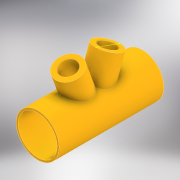
# Autodesk Inventor part: JuntaEjeCadera
Saved by Autodesk Inventor 2021 (Build 250183000, 183)
## iProperties
Created: 2024-02-21
Part Number: JuntaEjeCadera
Material: PLA
Document SubType Name: Modeling
Designer: Martin
Density: 1.27 g/cm^3
Appearance: PLA
Mass: 57.2544 g
Surface Area: 319.514 cm^2
Volume: 45.0822 cm^3
Author: Martin
Autodesk Inventor part; units mm, degrees
ref_plane "YZ Plane" through (0, 0, 0) normal (1, 0, 0) x (0, 1, 0)
ref_plane "XZ Plane" through (0, 0, 0) normal (0, 1, 0) x (-1, 0, 0)
ref_plane "XY Plane" through (0, 0, 0) normal (0, 0, 1) x (1, 0, 0)
sketch "Sketch1" plane through (0, 0, 0) normal (0, 0, 1) x (1, 0, 0)
  circle A0 centre (0, 0) radius 18.6
  circle A1 centre (0, 0) radius 20.5
  dimension "d0" = 37.2
  dimension "d1" = 41
  constraints: 2 centre point, 2 coincident
  measures "d0" diameter of A0
  measures "d1" diameter of A1
extrude "Extrusion1" add sketch "Sketch1" along normal blind 30
ref_plane "Work Plane1" through (0, 0, 0) normal (0, 1, 0) x (0, 0, 1)
ref_plane "Work Plane2" through (0, 40.5, 0) normal (0, 1, 0) x (0, 0, 1)
sketch "Sketch3" plane through (0, 0, 30) normal (0, 0, 1) x (1, 0, 0)
  circle A0 centre (0, 0) radius 20.5 projected
  circle A1 centre (0, 0) radius 18.6 projected
extrude "Extrusion3" add sketch "Sketch3" along normal blind 12
ref_plane "Work Plane3" through (0, 20.5, 0) normal (0, 1, 0) x (-1, 0, 0)
sketch "Sketch5" plane through (0, 40.5, 0) normal (0, 1, 0) x (0, 0, 1)
  line L0 (0, -20.5) -> (0, 20.5) projected
  line L1 (20, 20.5) -> (20, -20.5)
  point P0 (0, 0)
  dimension "d29" = 20
  constraints: 2 end point, 1 vertical
  measures "d29" distance between parallel lines of L0 L1
ref_plane "Work Plane4" through (20.5, 40.5, 20) normal (0, 0.9396926, 0.3420201) x (-1, 0, 0)
sketch "Sketch8" plane through (20.5, 40.5, 20) normal (0, 0.9396926, 0.3420201) x (-1, 0, 0)
  circle A0 centre (20.5, -1.2567) radius 12.5
  circle A1 centre (20.5, -1.2567) radius 7.9
  point P0 (20.5, -4.942)
  dimension "d44" = 25
  dimension "d45" = 15.8
  constraints: 2 centre point, 1 coincident
  measures "d44" diameter of A0
  measures "d45" diameter of A1
extrude "Extrusion6" add sketch "Sketch8" against normal up to surface round surface about axis through (0, 0, 0) along (0, 0, 1) radius 20.5 far side no
mirror "Mirror3" about plane through (0, 0, 0) normal (0, 0, 1) of "Extrusion1", "Extrusion6", "Extrusion3"
sketch "Sketch12" plane through (0, 0, -42) normal (0, 0, -1) x (-1, 0, 0)
  circle A0 centre (0, 0) radius 20.5 projected
  circle A1 centre (0, 0) radius 18.6 projected
  circle A2 centre (0, 0) radius 7.5
  line L0 (0, 3.5) -> (22, 3.5)
  line L1 (22, 3.5) -> (22, -3.5)
  line L2 (22, -3.5) -> (0, -3.5)
  line L3 (0, -3.5) -> (0, 3.5)
  line L4 (-29, 0) -> (30.5, 0) projected
  line L5 (0, 0) -> (5.3033, 5.3033)
  line L6 (0, 0) -> (7.5, 0) construction
  arc A3 (5.3033, 5.3033) -> (9.9668, 3.5) centre (11.1271, 13.4325) ccw
  line L7 (0, 0) -> (5.3033, -5.3033)
  arc A4 (9.9668, -3.5) -> (5.3033, -5.3033) centre (11.1271, -13.4325) ccw
  point P0 (20.199, -3.5)
  point P1 (20.199, 3.5)
  dimension "d50" = 15
  dimension "d51" = 22
  dimension "d52" = 7
  dimension "d53" = 3.5
  dimension "d54" = 3.5
  dimension "d55" = 45
  dimension "d56" = 5
  dimension "d57" = 10
  constraints: 14 end point, 4 point on circle, 3 symmetric about line, 2 centre point, 2 horizontal, 2 parallel, 1 coincident, 1 equal length, 1 perpendicular, 1 point on line, 4 other
  measures "d51" distance of L1.end L2.end
  measures "d52" distance of L0.end L1.end
  measures "d53" distance between parallel lines of L2 L4
  measures "d54" distance between parallel lines of L4 L0
  measures "d55" angle of L6 L5
  measures "d56" distance of L5.end A3.end
  measures "d57" radius of A3
extrude "Extrusion8" add sketch "Sketch12" along normal blind 10 contours L0 A1 L4 A0 | A0 L4 A1 L2 | L0 A3 A2 L4 A1 | A1 L4 A2 A4 L2 picked at (-19.4717, 3.1841) picked at (-19.4717, -3.1841)
sketch "Sketch15" plane through (0, 0, 42) normal (0, 0, 1) x (1, 0, 0)
  circle A0 centre (0, 0) radius 20.5 projected
  circle A1 centre (0, 0) radius 18.6 projected
extrude "Extrusion9" add sketch "Sketch15" along normal blind 6
sketch "Sketch16" plane through (0, 0, 0) normal (1, 0, 0) x (0, 1, 0)
  line L0 (45.2051, -7.0729) -> (36.6546, -30.5652) projected
  line L1 (36.6546, -30.5652) -> (20.5781, -30.5652)
  point P0 (0, 0)
  constraints: 2 end point, 1 horizontal
equation "\"d53\" = d54"
body "Solid1"
